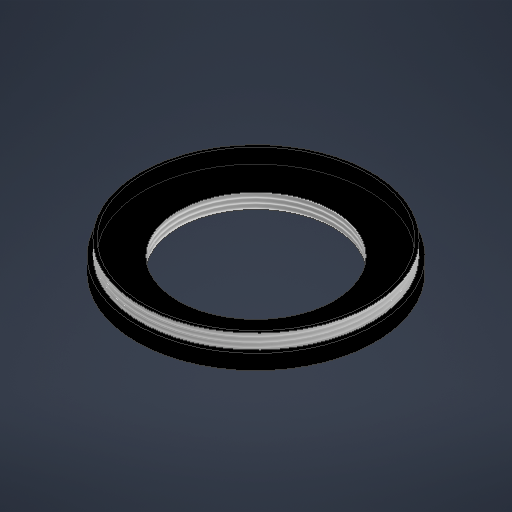
# Autodesk Inventor part: 77mm to 52mm
Saved by Autodesk Inventor 2026 (Build 300175000, 175)
## iProperties
Created: 2025-11-17
Part Number: 77mm to 52mm
Material: Aluminum 6061-AHC
Document SubType Name: Modeling
Designer: FiolkaLab
Mass: 41.9376 g
Surface Area: 101.568 cm^2
Volume: 15.5324 cm^3
Density: 2.7 g/cm^3
Appearance: Aluminum - Dark
Author: FiolkaLab
Autodesk Inventor part; units mm, degrees
ref_plane "YZ Plane" through (0, 0, 0) normal (1, 0, 0) x (0, 1, 0)
ref_plane "XZ Plane" through (0, 0, 0) normal (0, 1, 0) x (-1, 0, 0)
ref_plane "XY Plane" through (0, 0, 0) normal (0, 0, 1) x (1, 0, 0)
sketch "Sketch1" plane through (0, 0, 0) normal (0, 1, 0) x (-1, 0, 0)
  circle A0 centre (0, 0) radius 39.878
  dimension "d0" = 79.756
  constraints: 1 centre point, 1 coincident
  measures "d0" diameter of A0
extrude "Extrusion1" add sketch "Sketch1" along normal blind 5
sketch "Sketch2" plane through (0, 5, 0) normal (0, 1, 0) x (1, 0, 0)
  circle A0 centre (0, 0) radius 26
  dimension "d3" = 52
  constraints: 1 centre point, 1 coincident
  measures "d3" diameter of A0
extrude "Extrusion2" cut sketch "Sketch2" against normal blind 5
thread "Thread1" size "2 1/16-16 UNS" class "2B" standard "ANSI Unified Screw Threads" length 6.35
sketch "Sketch3" plane through (0, 5, 0) normal (0, 1, 0) x (1, 0, 0)
  circle A0 centre (0, 0) radius 38.5
  dimension "d8" = 77
  constraints: 1 centre point, 1 coincident
  measures "d8" diameter of A0
extrude "Extrusion3" add sketch "Sketch3" along normal blind 4.906
sketch "Sketch4" plane through (0, 9.906, 0) normal (0, 1, 0) x (1, 0, 0)
  circle A0 centre (0, 0) radius 37.5
  dimension "d11" = 75
  constraints: 1 centre point, 1 coincident
  measures "d11" diameter of A0
extrude "Extrusion4" cut sketch "Sketch4" against normal blind 4.906
thread "Thread3" size "3 1/8-16 UN" class "2A" standard "ANSI Unified Screw Threads" full length
body "Solid1"
